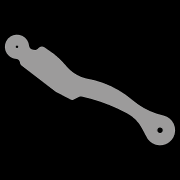
# Autodesk Inventor part: LowerLeg
Saved by Autodesk Inventor 2020 (Build 240168000, 168)
## iProperties
Created: 2020-05-17
Part Number: LowerLeg
Material: Generic
Document SubType Name: Sheet Metal
Designer: valer
Density: 1 g/cm^3
Sheet Metal Rule: Default
Appearance: Default
Author: valer
Autodesk Inventor part; units mm, degrees
ref_plane "YZ Plane" through (0, 0, 0) normal (1, 0, 0) x (0, 1, 0)
ref_plane "XZ Plane" through (0, 0, 0) normal (0, 1, 0) x (-1, 0, 0)
ref_plane "XY Plane" through (0, 0, 0) normal (0, 0, 1) x (1, 0, 0)
sketch "Base" plane through (0, 0, 0) normal (0, 0, 1) x (1, 0, 0)
  circle A0 centre (0, 0) radius 25.4
  arc A1 (257.1998, -154.5729) -> (134.8889, -104.8633) centre (59.6203, -465.39) ccw
  line L0 (6.0315, -24.6735) -> (7.0413, -37.3333)
  line L1 (-17.4625, -18.4451) -> (-13.314, -21.6309)
  line L2 (7.0413, -37.3333) -> (82.5854, -95.3476)
  line L3 (0, 0) -> (41.2806, -7.9386)
  line L4 (41.2806, -7.9386) -> (52.2222, 2.6699)
  line L5 (52.2222, 2.6699) -> (78.2666, -15.4892)
  arc A2 (105.165, -41.9173) -> (78.2666, -15.4892) centre (-46.5052, -169.3837) ccw
  arc A3 (105.165, -41.9173) -> (146.0514, -67.6944) centre (165.9303, 9.151) ccw
  arc A4 (245.7494, -113.8694) -> (146.0514, -67.6944) centre (113.6833, -268.2999) ccw
  arc A5 (245.7494, -113.8694) -> (311.6964, -146.808) centre (344.7991, 1.9534) ccw
  arc A6 (257.1998, -154.5729) -> (278.6053, -195.7416) centre (1107.1082, 261.1859) ccw
  arc A7 (328.9302, -198.4348) -> (311.6964, -146.808) centre (304.8, -177.8) ccw
  arc A8 (278.6053, -195.7416) -> (328.9302, -198.4348) centre (304.8, -177.8) ccw
  line L6 (82.5854, -95.3476) -> (116.796, -113.1736)
  line L7 (116.796, -113.1736) -> (118.4542, -112.9723)
  line L8 (118.4542, -112.9723) -> (117.4041, -113.4905)
  line L9 (110.9586, -117.0665) -> (110.7848, -117.0034)
  line L10 (82.5854, -95.3476) -> (82.8233, -95.4599)
  line L11 (6.0315, -24.6735) -> (0, 0)
  line L12 (117.4041, -113.4905) -> (134.8889, -104.8633)
  line L13 (134.8889, -104.8633) -> (133.3022, -96.2022)
  line L14 (82.8233, -95.4599) -> (81.0009, -83.9156)
  line L15 (133.3022, -96.2022) -> (123.4498, -86.7177)
  line L16 (90.8718, -73.9469) -> (103.6068, -78.9312)
  line L17 (81.0009, -83.9156) -> (90.8718, -73.9469)
  line L18 (104.6137, -82.5316) -> (117.3025, -87.4979)
  line L19 (123.4498, -86.7177) -> (117.3025, -87.4979)
  line L20 (106.4742, -88.8676) -> (100.0125, -89.6878)
  line L21 (103.6068, -78.9312) -> (104.6137, -82.5316)
  dimension "d0" = 50.8
  dimension "d1" = 12.7
  dimension "d2" = 95.25
  dimension "d3" = 42.037
  dimension "d4" = 15.24
  dimension "d5" = 31.75
  dimension "d6" = 198.12
  dimension "d7" = 79.375
  dimension "d8" = 203.2
  dimension "d9" = 38.5763
  dimension "d10" = 170
  dimension "d11" = 101
  dimension "d12" = 125
  dimension "d13" = 368.3
  dimension "d15" = 152.4
  dimension "d16" = 31.75
  dimension "d17" = 946.15
  dimension "d18" = 40.8864
  dimension "d19" = 304.8
  dimension "d20" = 177.8
  dimension "d21" = 165.9303
  dimension "d22" = 169.3837
  dimension "d23" = 154.5729
  dimension "d24" = 81.637
  dimension "d25" = 135.557
  dimension "d26" = 116.215
  dimension "d27" = 162.422
  dimension "d28" = 167.748
  dimension "d29" = 132.083
  dimension "d30" = 0.0558
  dimension "d31" = 153.7246
  dimension "d32" = 72.1956
  dimension "d33" = 906.7817
  dimension "d34" = 236.8783
  dimension "d35" = 68.2824
  dimension "d36" = 39.7668
  dimension "d45" = 127
  dimension "d46" = 42.096
  dimension "d47" = 6.388
  dimension "d48" = 16.148
  dimension "d49" = 135.244
  dimension "d50" = 97.195
  dimension "d51" = 43.507
  dimension "d52" = 2.9857
  dimension "d53" = 0.0046
  dimension "d54" = 113.7837
  dimension "d55" = 23.142
  dimension "d56" = 35.7403
  dimension "d57" = 101.5713
  dimension "d58" = 78.5187
  dimension "d59" = 19.6894
  dimension "d60" = 15.1033
  measures "d0" diameter of A0
  measures "d1" distance of L0.start L0.end
  measures "d2" distance of L0.end L2.end
  measures "d3" distance of L3.start L3.end
  measures "d4" distance of L3.end L4.end
  measures "d5" distance of L4.end L5.end
  measures "d6" radius of A2
  measures "d7" radius of A3
  measures "d8" radius of A4
  measures "d9" distance of L2.end L6.end
  measures "d10" angle of L6 L2
  measures "d11" angle of L5 L4
  measures "d12" angle of L4 L3
  measures "d13" radius of A1
  measures "d15" radius of A5
  measures "d16" radius of A7
  measures "d17" radius of A6
  measures "d18" horizontal distance of A2.start A3.end
  measures "d19" horizontal distance of point (0, 0) A7.centre
  measures "d20" vertical distance of A7.centre point (0, 0)
  measures "d21" horizontal distance of A3.centre point (0, 0)
  measures "d22" vertical distance of A2.centre point (0, 0)
  measures "d23" vertical distance of point (0, 0) A1.start
  measures "d24" angle of L4 L2
  measures "d25" angle of L7 L2
  measures "d26" angle of L8 L2
  measures "d27" angle of L9 L2
  measures "d28" angle of L10 L2
  measures "d29" angle of L0 L2
  measures "d30" distance between parallel lines of L1 L2
  measures "d31" distance from line of point (0, 0) L8
  measures "d32" distance from line of point (0, 0) L9
  measures "d33" distance from line of A6.centre L2
  measures "d34" distance from line of A5.centre L2
  measures "d35" distance from line of A7.start L2
  measures "d36" distance from line of A6.end L2
  measures "d45" angle of L21 L18
  measures "d46" angle of L13 L2
  measures "d47" angle of L15 L2
  measures "d48" angle of L16 L2
  measures "d49" angle of L19 L2
  measures "d50" angle of L17 L2
  measures "d51" angle of L14 L2
  measures "d52" distance between parallel lines of L18 L16
  measures "d53" distance between parallel lines of L20 L19
  measures "d54" distance from line of point (0, 0) L13
  measures "d55" distance from line of point (0, 0) L15
  measures "d56" distance from line of point (0, 0) L16
  measures "d57" distance from line of point (0, 0) L19
  measures "d58" distance from line of point (0, 0) L21
  measures "d59" distance from line of L20.start L2
  measures "d60" distance from line of L20.end L2
extrude "Plate1" add sketch "Base" along normal blind 5.08 contours A0 L3 L11 L1 | L3 L4 L5 A2 A3 A4 A5 A7 A8 A6 A1 L13 L15 L19 L18 L21 L16 L17 L14 L10 L2 L0 A0 | A0 L11 L3 | L10 L14 L17 L16 L21 L18 L19 L15 L13 L12 L7 L6
sketch "MountHoles" plane through (0, 0, 5.08) normal (0, 0, 1) x (1, 0, 0)
  arc A0 (278.6053, -195.7416) -> (311.6964, -146.808) centre (304.8, -177.8) ccw projected
  circle A1 centre (304.8, -177.8) radius 3.175
  circle A2 centre (0, 0) radius 3.175
  circle A3 centre (0, 0) radius 15.875 construction
  circle A4 centre (0, 15.875) radius 3.175
  line L0 (0, 15.875) -> (0, 0) construction
  circle A5 centre (-13.7482, 7.9375) radius 3.175
  circle A6 centre (-13.7482, -7.9375) radius 3.175
  circle A7 centre (0, -15.875) radius 3.175
  circle A8 centre (13.7482, -7.9375) radius 3.175
  circle A9 centre (13.7482, 7.9375) radius 3.175
  point P0 (14.9365, 6.9557)
  dimension "d40" = 31.75
  dimension "d38" = 6.35
  dimension "d39" = 6.35
  dimension "d43" = 360
  constraints: 8 centre point, 3 coincident, 2 end point, 1 equal radius, 1 vertical, 1 vertical alignment, 15 other
  measures "d38" diameter of A1
  measures "d39" diameter of A2
hole "MountHolesFeature" at (0, 0, 5.08) direction (0, 0, -1) diameter 6.35 end through all
fillet "SmallFilletsFeature" radius 8.89 8 edges at (41.2806, -7.9386, 2.54) (134.8889, -104.8633, 2.54) (116.796, -113.1736, 2.54) (82.5854, -95.3476, 2.54) (7.0413, -37.3333, 2.54) (24.943, -4.7967, 2.54) (6.0315, -24.6735, 2.54) (52.2222, 2.6699, 2.54)
fillet "LargeFilletsFeature" radius 76.2 1 edges at (257.1998, -154.5729, 2.54)
sketch "WheelMountHole" plane through (0, 0, 5.08) normal (0, 0, 1) x (1, 0, 0)
  arc A0 (278.6053, -195.7416) -> (311.6964, -146.808) centre (304.8, -177.8) ccw projected
  circle A1 centre (304.8, -177.8) radius 6.35
  point P0 (0, 0)
  dimension "d83" = 12.7
  constraints: 1 centre point, 1 coincident
  measures "d83" diameter of A1
hole "WheelMountHoleFeature" at (304.8, -177.8, 5.08) direction (0, 0, -1) diameter 12.7 end through all
sketch "ShockMountHole" plane through (0, 0, 5.08) normal (0, 0, 1) x (1, 0, 0)
  circle A0 centre (56.1234, -30.8576) radius 3.175 projected
  point P0 (0, 0)
hole "ShockMountHoleFeature" at (56.1234, -30.8576, 5.08) direction (0, 0, -1) diameter 6.35 end through all
equation "\"d66\" = Thickness"
equation "\"d89\" = Thickness"
equation "\"d96\" = Thickness"
equation "\"d37\" = Thickness"
equation "\"BendRadius\" = Thickness"
equation "\"BendReliefWidth\" = Thickness"
equation "\"BendReliefDepth\" = 0.5 * Thickness"
equation "\"CornerReliefSize\" = 4 * Thickness"
equation "\"MinimumRemnant\" = 2 * Thickness"
equation "\"TransitionRadius\" = BendRadius"
equation "\"JacobiRadiusSize\" = BendRadius"
equation "\"GapSize\" = Thickness"
equation "\"Thickness\" = 5.08"
body "Solid1"
